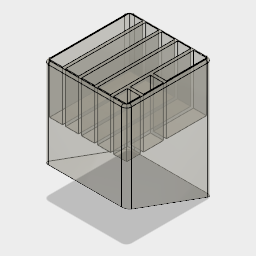
5_col_block (Autodesk Fusion 360 design; units mm, degrees)
Autodesk Fusion 360 part; units mm, degrees
sketch "Sketch1" plane through (0, 0, 0) normal (0, 1, 0) x (1, 0, 0)
  line L0 (41.5, 43) -> (-41.5, 43)
  line L1 (-41.5, 43) -> (-41.5, -43)
  line L2 (-41.5, -43) -> (41.5, -43)
  line L3 (41.5, -43) -> (41.5, 43)
  line L4 (41.5, 43) -> (-41.5, -43) construction
  line L5 (-41.5, 43) -> (41.5, -43) construction
  line L6 (-38.5, -39.8916) -> (-25.5, -39.8916)
  line L7 (-25.5, -39.8916) -> (-25.5, 40.1084)
  line L8 (-25.5, 40.1084) -> (-38.5, 40.1084)
  line L9 (-38.5, 40.1084) -> (-38.5, -39.8916)
  line L10 (-22.5, 40.1084) -> (-22.5, -39.8916)
  line L11 (-9.5, 40.1084) -> (-22.5, 40.1084)
  line L12 (-9.5, -39.8916) -> (-9.5, 40.1084)
  line L13 (-22.5, -39.8916) -> (-9.5, -39.8916)
  line L14 (-6.5, 40.1084) -> (-6.5, -39.8916)
  line L15 (6.5, 40.1084) -> (-6.5, 40.1084)
  line L16 (6.5, -39.8916) -> (6.5, 40.1084)
  line L17 (-6.5, -39.8916) -> (6.5, -39.8916)
  line L18 (9.5, 40.1084) -> (9.5, -39.8916)
  line L19 (22.5, 40.1084) -> (9.5, 40.1084)
  line L20 (22.5, -39.8916) -> (22.5, 40.1084)
  line L21 (9.5, -39.8916) -> (22.5, -39.8916)
  line L22 (38.5, 39.8916) -> (25.5, 39.8916)
  line L23 (25.5, 39.8916) -> (25.5, -0.1084)
  line L24 (25.5, -0.1084) -> (38.5, -0.1084)
  line L25 (38.5, -0.1084) -> (38.5, 39.8916)
  line L26 (38.5, -3.1084) -> (25.5, -3.1084)
  line L27 (25.5, -3.1084) -> (25.5, -23.1084)
  line L28 (25.5, -23.1084) -> (38.5, -23.1084)
  line L29 (38.5, -23.1084) -> (38.5, -3.1084)
  line L30 (38.5, -39.8916) -> (25.5, -39.8916)
  line L31 (25.5, -39.8916) -> (25.5, -26.1084)
  line L32 (25.5, -26.1084) -> (38.5, -26.1084)
  line L33 (38.5, -26.1084) -> (38.5, -39.8916)
  dimension "d1" = 83
  dimension "d2" = 86
  dimension "d3" = 80
  dimension "d4" = 13
  dimension "d5" = 3
  dimension "d8" = 48
  dimension "d9" = 0
  dimension "d10" = 3
  dimension "d11" = 40
  dimension "d12" = 3
  dimension "d13" = 3
  dimension "d14" = 20
  dimension "d17" = 13
  dimension "d18" = 3
  dimension "d19" = 3
  measures "d1" distance of L1.end L2.end
  measures "d2" distance of L0.start L2.end
  measures "d3" distance of L6.start L8.end
  measures "d4" distance of L6.start L6.end
  measures "d5" distance of L1 L9
  measures "d10" distance of L3 L25
  measures "d11" distance of L22.start L24.end
  measures "d12" distance of L24 L26
  measures "d13" distance of L3 L29
  measures "d14" distance of L26.start L28.end
  measures "d17" distance of L30.start L30.end
  measures "d18" distance of L3 L33
  measures "d19" distance of L28 L32
extrude "Extrude1" add sketch "Sketch1" along normal blind 70 contours L0 L1 L2 L3 | L6 L7 L8 L9 | L10 L11 L12 L13 | L14 L15 L16 L17 | L18 L19 L20 L21 | L22 L23 L24 L25 | L26 L27 L28 L29 | L30 L31 L32 L33
extrude "Extrude2" add sketch "Sketch1" along normal blind 50 from surface at 70
sketch "Sketch2" plane through (41.5, 0, 0) normal (1, 0, 0) x (0, 0, -1)
  line L0 (-43, 0) -> (43, 0)
  line L1 (43, 0) -> (43, 120)
  line L2 (43, 120) -> (-43, 120)
  line L3 (-43, 120) -> (-43, 0)
  line L4 (-43, 31.3014) -> (43, 0)
  dimension "d29" = 20
  measures "d29" angle of L0 L4
extrude "Extrude4" cut sketch "Sketch2" against normal up to surface (83 mm away) contours L0 L3 L4
fillet "Fillet2" radius 5 4 edges at (41.5, 75.6507, 43) (-41.5, 75.6507, 43) (41.5, 60, -43) (-41.5, 60, -43)
fillet "Fillet3" radius 2 8 edges at (40.0355, 120, 41.5355) (41.5, 120, 0) (40.0355, 120, -41.5355) (0, 120, -43) (-40.0355, 120, -41.5355) (-41.5, 120, 0) (-40.0355, 120, 41.5355) (0, 120, 43)
equation "d1 = ( ( 13 + 3 ) * 5 ) * 1 mm + 3 mm"
equation "d2 = 80 mm + 6 mm"
equation "d8 = ( 16 * 3 ) * 1 mm"
